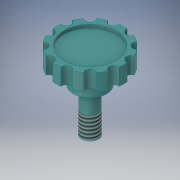
# Autodesk Inventor part: Lopez_Knob
Saved by Autodesk Inventor 2018 (Build 220112000, 112)
## iProperties
Created: 2018-02-08
Part Number: Lopez_Knob
Material: Polypropylene
Document SubType Name: Modeling
Designer: clopez06
Density: 0.899 g/cm^3
Appearance: Smooth - Ash
Author: clopez06
Autodesk Inventor part; units mm, degrees
ref_plane "YZ Plane" through (0, 0, 0) normal (1, 0, 0) x (0, 1, 0)
ref_plane "XZ Plane" through (0, 0, 0) normal (0, 1, 0) x (-1, 0, 0)
ref_plane "XY Plane" through (0, 0, 0) normal (0, 0, 1) x (1, 0, 0)
sketch "Sketch1" plane through (0, 0, 0) normal (0, 0, 1) x (1, 0, 0)
  line L0 (0, 0) -> (0, 29.21)
  line L1 (0, 29.21) -> (-12.7, 29.21)
  line L2 (-12.7, 29.21) -> (-12.7, 22.86)
  line L3 (-12.7, 22.86) -> (-6.35, 22.86)
  line L4 (-6.35, 22.86) -> (-6.35, 16.51)
  line L5 (-6.35, 16.51) -> (-3.175, 16.51)
  line L6 (-3.175, 16.51) -> (-3.175, 0)
  line L7 (-3.175, 0) -> (0, 0)
  dimension "d0" = 29.21
  dimension "d1" = 12.7
  dimension "d2" = 6.35
  dimension "d3" = 6.35
  dimension "d4" = 6.35
  dimension "d5" = 3.175
  constraints: 16 end point, 5 perpendicular, 2 vertical, 1 horizontal
  measures "d0" distance of L0.start L0.end
  measures "d1" distance of L0.end L1.end
  measures "d2" distance of L1.end L2.end
  measures "d3" distance of L2.end L3.end
  measures "d4" distance of L3.end L4.end
  measures "d5" distance of L4.end L5.end
revolve "Revolution1" add sketch "Sketch1" angle 360 about axis through (0, 0, 0) along (0, 1, 0)
sketch "Sketch2" plane through (0, 29.21, 0) normal (0, 1, 0) x (1, 0, 0)
  circle A0 centre (0, 0) radius 9.906
  dimension "d7" = 19.812
  constraints: 1 centre point, 1 coincident
  measures "d7" diameter of A0
sketch "Sketch3" plane through (0, 29.21, 0) normal (0, 1, 0) x (1, 0, 0)
  line L0 (0, 0) -> (-3.287, 12.2673)
  line L1 (0, 0) -> (0, 12.62)
  dimension "d8" = 12.7
  dimension "d9" = 15
  constraints: 4 end point, 1 vertical
  measures "d8" distance of L0.start L0.end
  measures "d9" angle of L1 L0
hole "Hole1" at (-3.287, 29.21, -12.2673) direction (0, -1, 0) diameter 3.556 end through all
pattern_circular "Circular Pattern1" count 12 over 360 about axis through (0, 26.035, 0) along (0, 1, 0) of "Hole1"
hole "Hole2" at (0, 29.21, 0) direction (0, -1, 0) diameter 19.812 depth 1.27
thread "Thread1" size "1/4-20 UNC" class "2A" standard "ANSI Unified Screw Threads" length 25.4 offset 8.128
body "Solid1"
